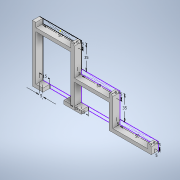
# Autodesk Inventor part: spicerack side
Saved by Autodesk Inventor 2020 (Build 240168000, 168)
## iProperties
Created: 2020-05-19
Part Number: spicerack side
Material: Generic
Document SubType Name: Modeling
Designer: maxde
Density: 1 g/cm^3
Appearance: Default
Author: maxde
Autodesk Inventor part; units mm, degrees
ref_plane "YZ Plane" through (0, 0, 0) normal (1, 0, 0) x (0, 1, 0)
ref_plane "XZ Plane" through (0, 0, 0) normal (0, 1, 0) x (-1, 0, 0)
ref_plane "XY Plane" through (0, 0, 0) normal (0, 0, 1) x (1, 0, 0)
sketch "Sketch1" plane through (0, 0, 0) normal (0, 0, 1) x (1, 0, 0)
  line L0 (-25, 3.3) -> (25, 3.3)
  line L1 (25, 3.3) -> (25, -3.3)
  line L2 (25, -3.3) -> (-25, -3.3)
  line L3 (-25, -3.3) -> (-25, 3.3)
  line L4 (-25, 3.3) -> (25, -3.3) construction
  line L5 (25, 3.3) -> (-25, -3.3) construction
  line L6 (25, 3.3) -> (30, 3.3)
  line L7 (30, 3.3) -> (30, -31.7)
  line L8 (30, -31.7) -> (25, -31.7)
  line L9 (25, -31.7) -> (25, 3.3)
  line L10 (30, -31.7) -> (80, -31.7)
  line L11 (80, -31.7) -> (80, -38.3)
  line L12 (80, -38.3) -> (30, -38.3)
  line L13 (30, -38.3) -> (30, -31.7)
  line L14 (30, -31.7) -> (80, -38.3) construction
  line L15 (80, -31.7) -> (30, -38.3) construction
  line L16 (25, -31.7) -> (30, -31.7)
  line L17 (30, -31.7) -> (30, -38.3)
  line L18 (30, -38.3) -> (25, -38.3)
  line L19 (25, -38.3) -> (25, -31.7)
  line L20 (-25, -3.3) -> (25, -3.3)
  line L21 (25, -3.3) -> (25, -8.3)
  line L22 (25, -8.3) -> (-25, -8.3)
  line L23 (-25, -8.3) -> (-25, -3.3)
  line L24 (25, -38.3) -> (80, -38.3)
  line L25 (80, -38.3) -> (80, -43.3)
  line L26 (80, -43.3) -> (25, -43.3)
  line L27 (25, -43.3) -> (25, -38.3)
  line L28 (80, -31.7) -> (85, -31.7)
  line L29 (85, -31.7) -> (85, -66.7)
  line L30 (85, -66.7) -> (80, -66.7)
  line L31 (80, -66.7) -> (80, -31.7)
  line L32 (85, -66.7) -> (135, -66.7)
  line L33 (85, -73.3) -> (85, -66.7)
  line L34 (135, -73.3) -> (85, -73.3)
  line L35 (135, -66.7) -> (135, -73.3)
  line L36 (85, -66.7) -> (135, -73.3) construction
  line L37 (135, -66.7) -> (85, -73.3) construction
  line L38 (80, -66.7) -> (85, -66.7)
  line L39 (85, -66.7) -> (85, -73.3)
  line L40 (85, -73.3) -> (80, -73.3)
  line L41 (80, -73.3) -> (80, -66.7)
  line L42 (80, -73.3) -> (135, -73.3)
  line L43 (135, -73.3) -> (135, -78.3)
  line L44 (135, -78.3) -> (80, -78.3)
  line L45 (80, -78.3) -> (80, -73.3)
  line L46 (135, -66.7) -> (140, -66.7)
  line L47 (140, -66.7) -> (140, -78.3)
  line L48 (140, -78.3) -> (135, -78.3)
  line L49 (135, -78.3) -> (135, -66.7)
  line L50 (-25, 3.3) -> (-30, 3.3)
  line L51 (-30, 3.3) -> (-30, -78.3)
  line L52 (-30, -78.3) -> (-25, -78.3)
  line L53 (-25, -78.3) -> (-25, 3.3)
  line L54 (-30, -78.3) -> (80, -78.3)
  line L55 (80, -78.3) -> (80, -73.3)
  line L56 (80, -73.3) -> (-30, -73.3)
  line L57 (-30, -73.3) -> (-30, -78.3)
  line L58 (25, -38.3) -> (30, -38.3)
  line L59 (30, -38.3) -> (30, -43.3)
  line L60 (30, -43.3) -> (25, -43.3)
  line L61 (25, -43.3) -> (25, -38.3)
  line L62 (25, -43.3) -> (30, -43.3)
  line L63 (30, -43.3) -> (30, -73.3)
  line L64 (30, -73.3) -> (25, -73.3)
  line L65 (25, -73.3) -> (25, -43.3)
  line L66 (-30, -78.3) -> (-15, -78.3)
  line L67 (-15, -78.3) -> (-15, -73.3)
  line L68 (-15, -73.3) -> (-30, -73.3)
  line L69 (-30, -73.3) -> (-30, -78.3)
  line L70 (30, -73.3) -> (15, -73.3)
  line L71 (15, -73.3) -> (15, -78.3)
  line L72 (15, -78.3) -> (30, -78.3)
  line L73 (30, -78.3) -> (30, -73.3)
  line L74 (25, -73.3) -> (40, -73.3)
  line L75 (40, -73.3) -> (40, -78.3)
  line L76 (40, -78.3) -> (25, -78.3)
  line L77 (25, -78.3) -> (25, -73.3)
  point P0 (0, 0)
  point P1 (-25, -73.3)
  dimension "d0" = 50
  dimension "d1" = 6.6
  dimension "d9" = 5
  dimension "d10" = 35
  dimension "d11" = 50
  dimension "d12" = 6.6
  dimension "d13" = 5
  dimension "d14" = 5
  dimension "d15" = 5
  dimension "d16" = 35
  dimension "d17" = 50
  dimension "d18" = 6.6
  dimension "d19" = 5
  dimension "d20" = 5
  dimension "d21" = 5
  dimension "d24" = 15
  dimension "d25" = 15
  dimension "d26" = 15
  constraints: 156 end point, 36 parallel, 18 horizontal, 18 perpendicular, 7 point on line, 2 midpoint
  measures "d0" distance of L1.end L2.end
  measures "d1" distance of L0.end L1.end
  measures "d9" distance of L7.end L8.end
  measures "d10" distance of L6.end L7.end
  measures "d11" distance of L12.start L13.start
  measures "d12" distance of L10.end L12.start
  measures "d13" distance of L20.end L21.end
  measures "d14" distance of L24.end L25.end
  measures "d15" distance of L30.start L41.end
  measures "d16" distance of L29.start L30.start
  measures "d17" distance of L34.start L33.start
  measures "d18" distance of L35.start L34.start
  measures "d19" distance of L42.end L44.start
  measures "d20" distance of L47.end L48.end
  measures "d21" distance of L52.end L51.end
  measures "d24" distance of L68.end L67.end
  measures "d25" distance of L72.end L71.end
  measures "d26" distance of L75.end L76.end
extrude "Extrusion1" add sketch "Sketch1" along normal blind 10 contours L3 L23 L53 L56 L51 L50 | L6 L7 L8 L9 L1 | L2 L9 L22 L23 | L56 L53 L52 L51 | L13 L18 L19 L8 | L56 L67 L54 L53 | L28 L29 L30 L31 L25 L11 | L59 L26 L27 L18 | L12 L25 L26 L59 | L63 L56 L65 L26 | L56 L77 L54 L71 | L33 L40 L41 L30 | L73 L54 L77 L56 | L56 L75 L54 L73 | L46 L47 L48 L43 L35 | L34 L43 L44 L45 L40
chamfer "Chamfer1" distance 2 angle 45 3 edges at (85, -31.7, 5) (30, 3.3, 5) (140, -66.7, 5)
body "Solid1"
